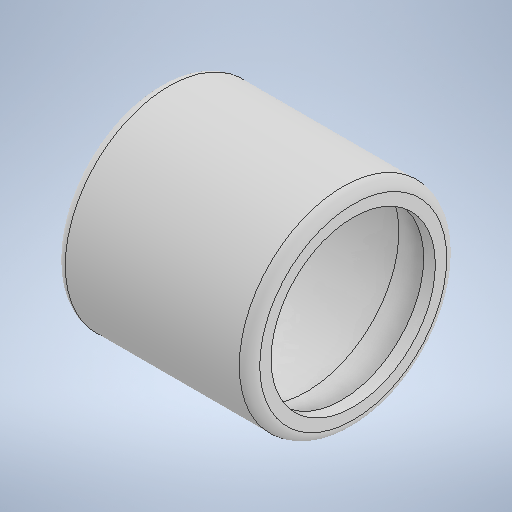
# Autodesk Inventor part: HFL2530_OutRing
Saved by Autodesk Inventor 2025.2 (Build 292293000, 293)
## iProperties
Created: 2024-11-28
Part Number: HFL2530_OutRing
Material: Generic
Document SubType Name: Modeling
Designer: Zvonko.Gabric
Density: 1 g/cm^3
Appearance: Default
Author: Zvonko.Gabric
Autodesk Inventor part; units mm, degrees
ref_plane "YZ Plane" through (0, 0, 0) normal (1, 0, 0) x (0, 1, 0)
ref_plane "XZ Plane" through (0, 0, 0) normal (0, 1, 0) x (-1, 0, 0)
ref_plane "XY Plane" through (0, 0, 0) normal (0, 0, 1) x (1, 0, 0)
sketch "Sketch1" plane through (0, 0, 0) normal (0, 1, 0) x (-1, 0, 0)
  line L0 (1.975, 1.575) -> (7.2, 1.575)
  line L1 (1.8, 0) -> (1.8, 1.4)
  line L2 (0, 0) -> (1.8, 0)
  line L3 (0, 1.75) -> (0, 0)
  line L4 (28.425, 3.325) -> (1.575, 3.325)
  line L5 (30, 0) -> (30, 1.75)
  line L6 (28.2, 0) -> (30, 0)
  line L7 (28.2, 2.205) -> (28.2, 0)
  line L8 (22.8, 2.205) -> (27.71, 2.205)
  line L9 (22.8, 1.9285) -> (22.8, 2.205)
  line L10 (7.2, 1.9285) -> (22.8, 1.9285)
  line L11 (7.2, 1.575) -> (7.2, 1.9285)
  arc A0 (1.975, 1.575) -> (1.8, 1.4) centre (1.975, 1.4) ccw
  arc A1 (1.575, 3.325) -> (0, 1.75) centre (1.575, 1.75) ccw
  arc A2 (30, 1.75) -> (28.425, 3.325) centre (28.425, 1.75) ccw
  arc A3 (28.2, 2.205) -> (27.71, 2.205) centre (27.955, 2.205) ccw
  line L12 (30, -12.675) -> (0.4613, -12.675) construction
  point P0 (30, 0.875)
  dimension "d0" = 0
  dimension "d1" = 1.8
  dimension "d2" = 1.75
  dimension "d3" = 3.325
  dimension "d4" = 1.575
  dimension "d5" = 1.4
  dimension "d6" = 0.175
  dimension "d7" = 30
  dimension "d8" = 26.85
  dimension "d9" = 1.75
  dimension "d10" = 1.8
  dimension "d11" = 0.245
  dimension "d12" = 4.91
  dimension "d13" = 15.6
  dimension "d14" = 5.225
  dimension "d15" = 0.3535
  dimension "d16" = 0.2765
  dimension "d17" = 2.205
  dimension "d18" = 1.575
  dimension "d19" = 12.675
  constraints: 26 end point, 8 point on circle, 4 centre point, 1 horizontal, 1 midpoint
  measures "d0" distance of point (0, 0) L2.start
  measures "d1" distance of L2.start L1.start
  measures "d2" distance of L3.start L2.start
  measures "d3" distance between parallel lines of L4 L2
  measures "d4" radius of A1
  measures "d5" distance of L1.start L1.end
  measures "d6" radius of A0
  measures "d7" distance from line of point (30, 0.875) L3
  measures "d8" distance of L4.start L4.end
  measures "d9" distance of L5.start L5.end
  measures "d10" distance of L6.start L5.start
  measures "d11" radius of A3
  measures "d12" distance of L8.start L8.end
  measures "d13" distance of L10.start L9.start
  measures "d14" distance of L0.start L0.end
  measures "d15" distance of L0.end L10.start
  measures "d16" distance of L9.start L8.start
  measures "d17" distance of L7.start L6.start
  measures "d18" radius of A2
  measures "d19" distance between parallel lines of L12 L2
revolve "Revolution1" add sketch "Sketch1" angle 360 about axis through (-30, 0, -12.675) along (1, 0, 0)
body "Solid1"
